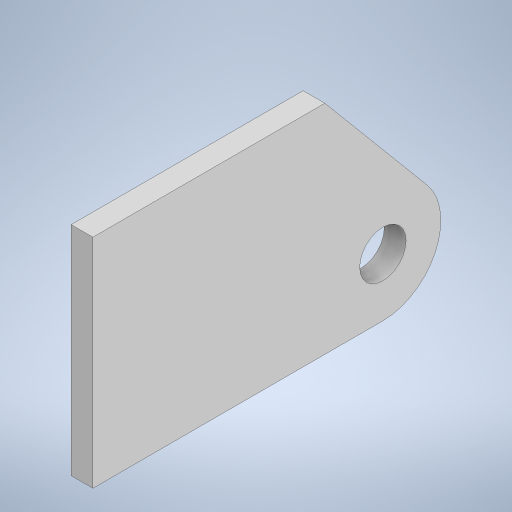
# Autodesk Inventor part: battery_cover_setter_joint
Saved by Autodesk Inventor 2024.1 (Build 281209000, 209)
## iProperties
Created: 2024-10-11
Part Number: battery_cover_setter_joint
Material: 一般
Document SubType Name: Sheet Metal
Designer: hibik
Density: 1 g/cm^3
Sheet Metal Rule: Default_mm
Appearance: 既定
Author: hibik
Autodesk Inventor part; units mm, degrees
ref_plane "YZ Plane" through (0, 0, 0) normal (1, 0, 0) x (0, 1, 0)
ref_plane "XZ Plane" through (0, 0, 0) normal (0, 1, 0) x (-1, 0, 0)
ref_plane "XY Plane" through (0, 0, 0) normal (0, 0, 1) x (1, 0, 0)
sketch "スケッチ1" plane through (0, 0, 0) normal (1, 0, 0) x (0, 1, 0)
  line L0 (0, 0) -> (15, 0)
  line L1 (15, 0) -> (15, -16)
  line L2 (15, -16) -> (0, -16)
  line L3 (0, -16) -> (0, 0)
  circle A0 centre (4, -20) radius 4
  circle A1 centre (4, -20) radius 1.6
  line L4 (15, -16) -> (6.5693, -23.0657)
  line L5 (0, -20) -> (0, -16)
  dimension "d0" = 15
  dimension "d2" = 3.2
  dimension "d3" = 8
  dimension "d5" = 20
  measures "d0" distance of L1.end L2.end
  measures "d2" diameter of A1
  measures "d3" diameter of A0
  measures "d5" distance from line of L0 A0.centre
extrude "プレート1" add sketch "スケッチ1" along normal blind 1.5
equation "\"d4\" = Thickness"
equation "\"BendRadius\" = Thickness"
equation "\"BendReliefWidth\" = Thickness"
equation "\"BendReliefDepth\" = 0.5 * Thickness"
equation "\"CornerReliefSize\" = 4 * Thickness"
equation "\"MinimumRemnant\" = 2 * Thickness"
equation "\"TransitionRadius\" = BendRadius"
equation "\"JacobiRadiusSize\" = BendRadius"
equation "\"GapSize\" = Thickness"
equation "\"Thickness\" = 1.5"
